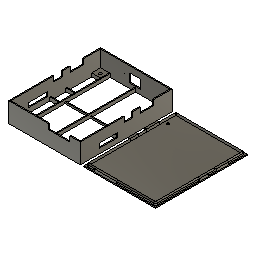
8x MP3 Platine (Autodesk Fusion 360 design; units mm, degrees)
Autodesk Fusion 360 part; units mm, degrees
box "Grundkörper Quader1" add length 104.4 width 81.4 height 21.6 placed x (0, 1, 0) y (-1, 0, 0) z (0, 0, 1) at (81.4, 0, 0) makes body 1
shell "Schale1" thickness 1.2 removed faces 1 at (27.1333, 34.8, 21.6) on bodies 1
extrude "Extrusion1" cut 1 faces at (27.5333, 35.2, 1.2) along direction (0, 0, -1) blind 1.2 on bodies 1 bodies 1
box "Grundkörper Quader2" add length 4 width 10 height 10 placed x (0, 0, 1) y (0, -1, 0) z (1, 0, 0) at (1.2, 11.2, 0) separate body makes body 2
cylinder "Grundkörper Zylinder1" add diameter 3 height -5 placed x (0, 1, 0) y (1, 0, 0) z (0, 0, -1) at (1.2, 1.2, 0) separate body makes body 3
pattern_linear "R-Anordnung1" count 2 spacing 90 along (0, 1, 0) of bodies 3 makes body 4
pattern_linear "R-Anordnung2" count 2 spacing 67 along (1, 0, 0) of bodies 4 3 makes body 5 at (68.713, -0.2095, 3.3333) makes body 6 at (68.713, 92.6095, 3.3333)
move_body "Verschieben1" bodies 6 3 4 5 to x (1, 0, 0) y (0, 1, 0) z (0, 0, 1) at (6, 0, 0)
move_body "Verschieben2" bodies 6 3 4 5 to x (1, 0, 0) y (0, 1, 0) z (0, 0, 1) at (0, 6, 0)
copy_body "Körper kopieren/einfügen1" bodies 2 makes body 7
move_body "Verschieben3" bodies 7 to x (1, 0, 0) y (0, 1, 0) z (0, 0, 1) at (69, 0, 0)
copy_body "Körper kopieren/einfügen2" bodies 7 2 makes body 8 makes body 9
move_body "Verschieben4" bodies 8 9 to x (1, 0, 0) y (0, 1, 0) z (0, 0, 1) at (0, 92, 0)
fillet "Abrundung1" radius 3 4 edges at (11.2, 11.2, 2) (70.2, 11.2, 2) (70.2, 93.2, 2) (11.2, 93.2, 2) on bodies 2 7 8 9
combine "Kombinieren1" operation cut target body 2 tool bodies 3
combine "Kombinieren2" operation cut target body 9 tool bodies 4
combine "Kombinieren3" operation cut target body 7 tool bodies 5
combine "Kombinieren4" operation cut target body 8 tool bodies 6
box "Grundkörper Quader3" add length 5 width 11 height -5 placed x (0, 0, 1) y (-1, 0, 0) z (0, -1, 0) at (41.1282, 103.2, 7.0845) separate body makes body 10
move_body "Verschieben5" bodies 10 to x (1, 0, 0) y (0, 1, 0) z (0, 0, 1) at (40.2718, 0, 0)
move_body "Verschieben6" bodies 10 to x (1, 0, 0) y (0, 1, 0) z (0, 0, 1) at (0, 0, -7.0845)
move_body "Verschieben7" bodies 10 to x (1, 0, 0) y (0, 1, 0) z (0, 0, 1) at (0, 0, 5.6)
move_body "Verschieben8" bodies 10 to x (1, 0, 0) y (0, 1, 0) z (0, 0, 1) at (-35.2, 0, 0)
combine "Kombinieren5" operation cut target body 1 tool bodies 10
box "Grundkörper Quader4" add length 5 width 25 height -5 placed x (0, 0, 1) y (1, 0, 0) z (0, 1, 0) at (55.2, 1.2, 10.3705) separate body makes body 11
move_body "Verschieben9" bodies 11 to x (1, 0, 0) y (0, 1, 0) z (0, 0, 1) at (-10.5, 0, 0)
move_body "Verschieben10" bodies 11 to x (1, 0, 0) y (0, 1, 0) z (0, 0, 1) at (0, 0, 6.2295)
combine "Kombinieren6" operation cut target body 1 tool bodies 11
box "Grundkörper Quader5" add length 5 width 21 height -5 placed x (0, 0, -1) y (0, -1, 0) z (-1, 0, 0) at (80.2, 22.2, 9.5461) separate body makes body 12
move_body "Verschieben11" bodies 12 to x (1, 0, 0) y (0, 1, 0) z (0, 0, 1) at (0, 0, 1.054)
move_body "Verschieben12" bodies 12 to x (1, 0, 0) y (0, 1, 0) z (0, 0, 1) at (0, 20.6, 0)
move_face "Flächen versetzen1" offset 99 1 faces at (80.2, 35.8, 8.9334) on bodies 12
combine "Kombinieren7" operation cut target body 1 tool bodies 12
box "Grundkörper Quader6" add length 10 width 91 height -5 placed x (0, 1, 0) y (-1, 0, 0) z (0, 0, 1) at (86, 45, 21.6) separate body makes body 13
move_body "Verschieben13" bodies 13 to x (1, 0, 0) y (0, 1, 0) z (0, 0, 1) at (0, -43.8, 0)
move_body "Verschieben14" bodies 13 to x (1, 0, 0) y (0, 1, 0) z (0, 0, 1) at (0, 43.25, 0)
move_body "Verschieben15" bodies 13 to x (1, 0, 0) y (0, 1, 0) z (0, 0, 1) at (0, 5.5, 0)
copy_body "Körper kopieren/einfügen3" bodies 13 makes body 14
move_body "Verschieben16" bodies 14 to x (1, 0, 0) y (0, 1, 0) z (0, 0, 1) at (0, 24, 0)
move_face "Flächen versetzen2" offset 5 1 faces at (55.6667, 73.95, 18.2667) on bodies 14
move_body "Verschieben17" bodies 14 to x (1, 0, 0) y (0, 1, 0) z (0, 0, 1) at (0, 19.25, 0)
move_body "Verschieben18" bodies 14 to x (1, 0, 0) y (0, 1, 0) z (0, 0, 1) at (0, -19.5, 0)
combine "Kombinieren8" operation cut target body 1 tool bodies 14 13
box "Grundkörper Quader7" add length 102.8 width 1.2 height -4 placed x (0, -1, 0) y (-1, 0, 0) z (0, 0, -1) at (40.2, 104, 0) separate body makes body 15
move_body "Verschieben19" bodies 15 to x (1, 0, 0) y (0, 1, 0) z (0, 0, 1) at (0.8, -0.2, 0)
box "Grundkörper Quader8" add length 1.2 width 38.8 height -4 placed x (0, -1, 0) y (-1, 0, 0) z (0, 0, -1) at (40, 91.4396, 0) separate body makes body 16
copy_body "Körper kopieren/einfügen4" bodies 15 makes body 17
move_body "Verschieben20" bodies 17 to x (1, 0, 0) y (0, 1, 0) z (0, 0, 1) at (-29, 0, 0)
copy_body "Körper kopieren/einfügen5" bodies 15 makes body 18
move_body "Verschieben21" bodies 18 to x (1, 0, 0) y (0, 1, 0) z (0, 0, 1) at (29, 0, 0)
move_body "Verschieben22" bodies 17 to x (1, 0, 0) y (0, 1, 0) z (0, 0, 1) at (0.4, 0, 0)
delete_face "Fläche löschen1" 1 faces at (9.7, 93.6019, 1.3333) on bodies 9
delete_face "Fläche löschen2" 1 faces at (71.0288, 94.1298, 1.3333) on bodies 8
delete_face "Fläche löschen3" 1 faces at (71.0288, 10.2702, 1.3333) on bodies 7
delete_face "Fläche löschen4" 1 faces at (11.1966, 8.3427, 1.3333) on bodies 2
move_body "Verschieben23" bodies 18 to x (1, 0, 0) y (0, 1, 0) z (0, 0, 1) at (0.2, 0, 0)
move_face "Flächen versetzen3" offset -5 1 faces at (42.5333, 104, 10.6) on bodies 1
move_face "Flächen versetzen4" offset -0.5 2 faces at (35.2, 104, 12.2667) (46.2, 104, 12.2667) on bodies 1
box "Grundkörper Quader9" add length 104.4 width 81.4 height 1.2 placed x (0, 1, 0) y (-1, 0, 0) z (0, 0, 1) at (81.4, 0, 21.6) separate body makes body 19
box "Grundkörper Quader10" add length 101.8 width 78.8 height -3 placed x (0, 1, 0) y (-1, 0, 0) z (0, 0, 1) at (80, 1.2, 21.6) separate body makes body 20
move_body "Verschieben24" bodies 20 to x (1, 0, 0) y (0, 1, 0) z (0, 0, 1) at (0.1, 0.1, 0)
fillet "Abrundung2" radius 2 4 edges at (80.1, 103.1, 20.1) (1.3, 103.1, 20.1) (1.3, 1.3, 20.1) (80.1, 1.3, 20.1) on bodies 20
shell "Schale2" thickness 1.2 removed faces 1 at (53.8333, 68.5, 21.6) on bodies 20
extrude "Extrusion2" cut 1 faces at (53.4333, 68.5, 19.8) along direction (0, 0, -1) blind 1.2 on bodies 20 bodies 20
chamfer "Fase1" distance 1.2 distance2 1.2 8 edges at (79.5142, 102.5142, 18.6) (40.7, 103.1, 18.6) (1.8858, 102.5142, 18.6) (1.3, 52.2, 18.6) (1.8858, 1.8858, 18.6) (40.7, 1.3, 18.6) (79.5142, 1.8858, 18.6) (80.1, 52.2, 18.6) measured on face at (80.0639, 101.4785, 19.6) measured on face at (79.3, 35.9, 18.6) measured on face at (1.8525, 102.4802, 19.6) measured on face at (79.3, 35.9, 18.6) measured on face at (2.0637, 1.7279, 19.6) measured on face at (79.3, 35.9, 18.6) measured on face at (79.5475, 1.9198, 19.6) measured on face at (79.3, 35.9, 18.6) on bodies 20
cylinder "Grundkörper Zylinder2" add diameter 3 height -5 placed x (1, 0, 0) y (0, 1, 0) z (0, 0, 1) at (74.7703, 89.2524, 22.8) separate body makes body 21
move_body "Verschieben25" bodies 21 to x (1, 0, 0) y (0, 1, 0) z (0, 0, 1) at (-0.0306, -0.0245, 0)
combine "Kombinieren9" operation cut target body 19 tool bodies 21
chamfer "Fase2" distance 1.2 distance2 1.2 1 edges at (74.1972, 87.8294, 22.8) measured on face at (24.5302, 64.2212, 22.8) on bodies 19
sketch "Skizze13" plane through (0, 104.4, 0) normal (0, 1, 0) x (-1, 0, 0)
  line L0 (-46.7, 5.6) -> (-46.7, 15.6)
  line L1 (-46.7, 15.6) -> (-34.7, 15.6)
  line L2 (-34.7, 15.6) -> (-34.7, 5.6)
  line L3 (-34.7, 5.6) -> (-46.7, 5.6)
  line L4 (-81.4, 21.6) -> (-81.4, 0)
  line L5 (-81.4, 0) -> (0, 0)
  line L6 (0, 0) -> (0, 21.6)
  line L7 (0, 21.6) -> (-81.4, 21.6)
  line L8 (-57.6244, 5.277) -> (-45.6244, 5.277) construction
  line L9 (-45.6244, 5.277) -> (-45.6244, 14.277) construction
  line L10 (-45.6244, 14.277) -> (-57.6244, 14.277) construction
  line L11 (-57.6244, 14.277) -> (-57.6244, 5.277) construction
  line L12 (-31.446, -0.4413) -> (-18.446, -0.4413) construction
  line L13 (-18.446, -0.4413) -> (-18.446, 11.5587) construction
  line L14 (-18.446, 11.5587) -> (-31.446, 11.5587) construction
  line L15 (-31.446, 11.5587) -> (-31.446, -0.4413) construction
  dimension "d81" = 10
  dimension "d82" = 10
  text T0 "+" font "Arial" height 10 bold align left top in box 12 x 9 at (-57.6244, 5.277) x (1, 0) y (0, 1) spacing 1 kerned
  text T1 "–" font "Arial" height 10 bold align left top in box 13 x 12 at (-31.446, -0.4413) x (1, 0) y (0, 1) spacing 1 kerned
extrude "Extrusion3" cut sketch "Skizze13" against normal blind 0.4 text T0 T1 bodies 1
extrude "Extrusion4" add 2 faces at (0.4, 73.7, 16.6) (0.4, 53.2833, 16.6) along direction (0, 0, 1) blind 3 separate body on bodies 1 makes body 22 at (0, 73.7, 17.6) makes body 23 at (0, 53.2833, 17.6)
move_body "Verschieben26" bodies 22 23 to x (1, 0, 0) y (0, 1, 0) z (0, 0, 1) at (0, 0, 2)
move_body "Verschieben27" bodies 22 23 to x (1, 0, 0) y (0, 1, 0) z (0, 0, 1) at (0, -0.2, 0)
move_face "Flächen versetzen5" offset -0.4 2 faces at (0.8, 68.5, 19.6) (0.8, 49.75, 19.6) on bodies 22 23
copy_body "Körper kopieren/einfügen6" bodies 23 22 makes body 24 makes body 25
move_body "Verschieben28" bodies 24 25 to x (1, 0, 0) y (0, 1, 0) z (0, 0, 1) at (80.1, 0, 0)
move_body "Verschieben29" bodies 24 25 to x (1, 0, 0) y (0, 1, 0) z (0, 0, 1) at (0.1, 0, 0)
move_face "Flächen versetzen6" offset 1.3 2 faces at (80.2, 53.35, 19.6) (80.2, 73.7667, 19.6) on bodies 24 25
move_face "Flächen versetzen7" offset 1.3 2 faces at (1.2, 73.7667, 19.6) (1.2, 53.35, 19.6) on bodies 22 23
extrude "Extrusion5" add 1 faces at (53.0333, 0.4, 16.6) along direction (0, 0, 1) blind 3 separate body on bodies 1 makes body 26
move_body "Verschieben30" bodies 26 to x (1, 0, 0) y (0, 1, 0) z (0, 0, 1) at (-0.2, 0, 0)
move_face "Flächen versetzen8" offset -0.4 1 faces at (44.5, 0.4, 17.6) on bodies 26
move_body "Verschieben31" bodies 26 to x (1, 0, 0) y (0, 1, 0) z (0, 0, 1) at (0, 0, 2)
move_face "Flächen versetzen9" offset 1.3 1 faces at (53.1, 1.2, 19.6) on bodies 26
move_body "Verschieben32" bodies 19 22 23 25 20 26 24 to x (-1, 0, 0) y (0, 1, 0) z (0, 0, -1) at (167, 0, 22.8)
box "Grundkörper Quader11" add length 1.2 width 10 height -4 placed x (0, 1, 0) y (1, 0, 0) z (0, 0, -1) at (70.2, 42.7181, 0) separate body makes body 27
move_body "Verschieben33" bodies 27 to x (1, 0, 0) y (0, 1, 0) z (0, 0, 1) at (0, 3, 0)
copy_body "Körper kopieren/einfügen7" bodies 27 makes body 28
move_body "Verschieben34" bodies 28 to x (1, 0, 0) y (0, 1, 0) z (0, 0, 1) at (0, 18, 0)
copy_body "Körper kopieren/einfügen8" bodies 28 27 makes body 29 makes body 30
move_body "Verschieben35" bodies 29 30 to x (1, 0, 0) y (0, 1, 0) z (0, 0, 1) at (-69, 0, 0)
copy_body "Körper kopieren/einfügen9" bodies 30 makes body 31
move_body "Verschieben36" bodies 31 to x (1, 0, 0) y (0, 1, 0) z (0, 0, 1) at (11.2, -12.7536, 0)
move_face "Flächen versetzen10" offset 32.6 1 faces at (22.4, 33.7645, 2.6667) on bodies 31
move_body "Verschieben37" bodies 31 to x (1, 0, 0) y (0, 1, 0) z (0, 0, 1) at (0, 0.1, 0)
extrude "Extrusion6" add 5 faces at (0.4, 17.05, 21.6) (81, 17.05, 21.6) (80.6, 62.8667, 21.6) (53.8667, 104, 21.6) (0.8, 62.8667, 21.6) along direction (0, 0, 1) blind 1 on bodies 1 bodies 1
move_body "Verschieben39" bodies 31 to x (1, 0, 0) y (0, 1, 0) z (0, 0, 1) at (14, 0, 0)
move_face "Flächen versetzen12" offset 14 1 faces at (26.4, 33.8645, 2.6667) on bodies 31
move_face "Flächen versetzen13" offset -2 1 faces at (50.1333, 33.4645, 4) on bodies 31
move_body "Verschieben40" bodies 31 to x (1, 0, 0) y (0, 1, 0) z (0, 0, 1) at (0, -31.8645, 0)
move_body "Verschieben41" bodies 31 to x (1, 0, 0) y (0, 1, 0) z (0, 0, 1) at (0, 50.4, 0)
box "Grundkörper Quader12" add length 10 width 36 height -2 placed x (0, 0, 1) y (1, 0, 0) z (0, 1, 0) at (10.7, 104.4, 5.6) separate body makes body 32
move_body "Verschieben42" bodies 32 to x (1, 0, 0) y (0, 1, 0) z (0, 0, 1) at (12, 0, 0)
copy_body "Körper kopieren/einfügen11" bodies 1 makes body 33
copy_body "Körper kopieren/einfügen12" bodies 32 makes body 34
combine "Kombinieren10" operation cut target body 1 tool bodies 34
combine "Kombinieren11" operation intersect target body 33 tool bodies 32 makes body 35 at (50.7, 103.2, 12.2667)
box "Grundkörper Quader13" add length 10 width 36 height -1 placed x (0, 0, 1) y (1, 0, 0) z (0, 1, 0) at (22.7, 104.4, 5.6) separate body makes body 36
move_body "Verschieben43" bodies 36 35 33 to x (-1, 0, 0) y (0, 1, 0) z (0, 0, -1) at (81.4, 0, 21.2)
combine "Kombinieren12" operation add target body 1 tool bodies 35 33
hidden bodies 16 36
equation "d65 = 102.00 mm - 0.2 mm"
equation "d66 = 79.00 mm - 0.2 mm"
named bodies: "Deckel", "Plus-Minus"
